Autodesk Fusion 360 part; units mm, degrees
note: some values were not read from the file. Set by a fixed rule: which sketch regions a step uses.
(part 5 of 15)
  line L3455 (261.579, -122.394) -> (261.6, -122.21)
  line L3456 (263.32, -121.881) -> (263.407, -122.045)
  line L3457 (42.9075, -121.723) -> (43.0718, -121.637)
  line L3458 (71.3052, -121.572) -> (71.4695, -121.486)
  line L3459 (70.8754, -122.354) -> (70.8961, -122.17)
  line L3460 (43.0718, -121.637) -> (43.2497, -121.585)
  line L3461 (282.196, -122.153) -> (282.03, -122.236)
  line L3462 (72.7572, -122.183) -> (72.7753, -122.367)
  line L3463 (42.5545, -122.144) -> (42.6438, -121.982)
  line L3464 (282.637, -121.35) -> (282.636, -121.377)
  line L3465 (282.342, -122.038) -> (282.196, -122.153)
  line L3466 (263.479, -122.407) -> (263.479, -122.434)
  line L3467 (72.1689, -123.253) -> (71.9903, -123.303)
  line L3468 (262.009, -121.612) -> (262.173, -121.526)
  line L3469 (71.0268, -122.882) -> (70.9421, -122.717)
  line L3470 (261.6, -122.21) -> (261.656, -122.033)
  line L3471 (72.0164, -121.437) -> (72.1935, -121.491)
  line L3472 (282.636, -121.377) -> (282.613, -121.561)
  line L3473 (261.745, -121.87) -> (261.864, -121.728)
  line L3474 (282.478, -120.825) -> (282.565, -120.988)
  line L3475 (72.4994, -121.698) -> (72.6166, -121.841)
  line L3476 (42.4984, -122.321) -> (42.5545, -122.144)
  line L3477 (72.775, -122.394) -> (72.7517, -122.578)
  line L3478 (72.4805, -123.055) -> (72.3344, -123.169)
  line L3479 (262.149, -123.278) -> (261.987, -123.187)
  line L3480 (262.873, -123.293) -> (262.694, -123.343)
  line L3481 (262.351, -121.474) -> (262.536, -121.457)
  line L3482 (71.8054, -123.317) -> (71.6213, -123.295)
  line L3483 (263.06, -121.62) -> (263.203, -121.738)
  line L3484 (72.3566, -121.58) -> (72.4994, -121.698)
  line L3485 (53.5942, -121.521) -> (53.5357, -121.697)
  line L3486 (53.3419, -120.641) -> (53.4591, -120.785)
  line L3487 (51.7946, -120.936) -> (51.8839, -120.774)
  line L3488 (52.3119, -120.43) -> (52.4898, -120.377)
  line L3489 (51.7845, -121.66) -> (51.7334, -121.482)
  line L3490 (70.8909, -122.539) -> (70.8754, -122.354)
  line L3491 (51.7386, -121.113) -> (51.7946, -120.936)
  line L3492 (52.8328, -122.246) -> (52.6479, -122.26)
  line L3493 (53.5357, -121.697) -> (53.4441, -121.858)
  line L3494 (301.464, -120.006) -> (301.607, -120.125)
  line L3495 (281.022, -120.672) -> (281.167, -120.556)
  line L3496 (52.6479, -122.26) -> (52.4638, -122.238)
  line L3497 (301.607, -120.125) -> (301.724, -120.268)
  line L3498 (282.555, -121.737) -> (282.463, -121.898)
  line L3499 (280.814, -120.976) -> (280.903, -120.814)
  line L3500 (52.8588, -120.38) -> (53.0359, -120.435)
  line L3501 (53.4591, -120.785) -> (53.5461, -120.948)
  line L3502 (281.693, -120.401) -> (281.878, -120.42)
  line L3503 (301.724, -120.268) -> (301.811, -120.432)
  line L3504 (301.864, -120.61) -> (301.882, -120.794)
  line L3505 (281.003, -122.01) -> (280.888, -121.865)
  line L3506 (282.218, -120.563) -> (282.361, -120.681)
  line L3507 (281.331, -120.47) -> (281.509, -120.417)
  line L3508 (51.7179, -121.297) -> (51.7386, -121.113)
  line L3509 (281.483, -122.278) -> (281.306, -122.221)
  line L3510 (51.8693, -121.825) -> (51.7845, -121.66)
  line L3511 (280.737, -121.337) -> (280.757, -121.153)
  line L3512 (52.1476, -120.515) -> (52.3119, -120.43)
  line L3513 (71.832, -121.417) -> (72.0164, -121.437)
  line L3514 (281.509, -120.417) -> (281.693, -120.401)
  line L3515 (280.752, -121.522) -> (280.737, -121.337)
  line L3516 (53.3229, -121.998) -> (53.1768, -122.113)
  line L3517 (280.803, -121.7) -> (280.752, -121.522)
  line L3518 (53.1768, -122.113) -> (53.0113, -122.196)
  line L3519 (52.0031, -120.632) -> (52.1476, -120.515)
  line L3520 (301.859, -121.005) -> (301.8, -121.18)
  line L3521 (53.0113, -122.196) -> (52.8328, -122.246)
  line L3522 (70.9421, -122.717) -> (70.8909, -122.539)
  line L3523 (281.167, -120.556) -> (281.331, -120.47)
  line L3524 (71.0415, -121.83) -> (71.1607, -121.688)
  line L3525 (281.145, -122.131) -> (281.003, -122.01)
  line L3526 (53.5461, -120.948) -> (53.5997, -121.126)
  line L3527 (52.2875, -122.181) -> (52.1256, -122.091)
  line L3528 (71.1607, -121.688) -> (71.3052, -121.572)
  line L3529 (53.6174, -121.337) -> (53.5942, -121.521)
  line L3530 (52.4898, -120.377) -> (52.6744, -120.36)
  line L3531 (280.903, -120.814) -> (281.022, -120.672)
  line L3532 (282.361, -120.681) -> (282.478, -120.825)
  line L3533 (53.6178, -121.31) -> (53.6174, -121.337)
  line L3534 (301.123, -119.863) -> (301.301, -119.918)
  line L3535 (281.306, -122.221) -> (281.145, -122.131)
  line L3536 (52.6744, -120.36) -> (52.8588, -120.38)
  line L3537 (281.667, -122.3) -> (281.483, -122.278)
  line L3538 (282.613, -121.561) -> (282.555, -121.737)
  line L3539 (52.1256, -122.091) -> (51.9844, -121.97)
  line L3540 (301.301, -119.918) -> (301.464, -120.006)
  line L3541 (51.7334, -121.482) -> (51.7179, -121.297)
  line L3542 (70.9522, -121.993) -> (71.0415, -121.83)
  line L3543 (280.757, -121.153) -> (280.814, -120.976)
  line L3544 (53.5997, -121.126) -> (53.6178, -121.31)
  line L3545 (53.0359, -120.435) -> (53.199, -120.523)
  line L3546 (280.888, -121.865) -> (280.803, -121.7)
  line L3547 (53.199, -120.523) -> (53.3419, -120.641)
  line L3548 (53.4441, -121.858) -> (53.3229, -121.998)
  line L3549 (301.442, -121.596) -> (301.276, -121.68)
  line L3550 (34.372, -120.754) -> (34.3717, -120.781)
  line L3551 (300.728, -121.722) -> (300.552, -121.665)
  line L3552 (301.811, -120.432) -> (301.864, -120.61)
  line L3553 (301.8, -121.18) -> (301.709, -121.342)
  line L3554 (52.4638, -122.238) -> (52.2875, -122.181)
  line L3555 (34.2133, -120.228) -> (34.3004, -120.392)
  line L3556 (300.577, -119.913) -> (300.754, -119.861)
  line L3557 (34.2899, -121.14) -> (34.1983, -121.302)
  line L3558 (299.983, -120.781) -> (300.003, -120.597)
  line L3559 (300.754, -119.861) -> (300.939, -119.844)
  line L3560 (300.39, -121.574) -> (300.249, -121.454)
  line L3561 (299.998, -120.966) -> (299.983, -120.781)
  line L3562 (300.913, -121.744) -> (300.728, -121.722)
  line L3563 (32.9018, -119.959) -> (33.0662, -119.873)
  line L3564 (33.587, -121.69) -> (33.4021, -121.704)
  line L3565 (32.5489, -120.38) -> (32.6382, -120.217)
  line L3566 (300.134, -121.309) -> (300.049, -121.144)
  line L3567 (34.0961, -120.085) -> (34.2133, -120.228)
  line L3568 (34.1983, -121.302) -> (34.0772, -121.442)
  line L3569 (32.6235, -121.269) -> (32.5387, -121.104)
  line L3570 (300.412, -119.999) -> (300.577, -119.913)
  line L3571 (199.319, -117.044) -> (199.582, -117.146)
  line L3572 (33.9311, -121.556) -> (33.7656, -121.64)
  line L3573 (33.4287, -119.804) -> (33.6131, -119.823)
  line L3574 (33.7902, -119.878) -> (33.9533, -119.966)
  line L3575 (301.097, -121.73) -> (300.913, -121.744)
  line L3576 (300.059, -120.42) -> (300.149, -120.257)
  line L3577 (200.711, -118.673) -> (200.731, -118.955)
  line L3578 (32.6382, -120.217) -> (32.7574, -120.075)
  line L3579 (300.552, -121.665) -> (300.39, -121.574)
  line L3580 (300.149, -120.257) -> (300.268, -120.115)
  line L3581 (200.419, -117.884) -> (200.553, -118.132)
  line L3582 (200.651, -118.397) -> (200.711, -118.673)
  line L3583 (33.244, -119.821) -> (33.4287, -119.804)
  line L3584 (301.276, -121.68) -> (301.097, -121.73)
  line L3585 (300.049, -121.144) -> (299.998, -120.966)
  line L3586 (34.3004, -120.392) -> (34.3539, -120.569)
  line L3587 (34.3484, -120.964) -> (34.2899, -121.14)
  line L3588 (301.882, -120.794) -> (301.882, -120.821)
  line L3589 (199.829, -117.284) -> (200.053, -117.455)
  line L3590 (199.043, -116.98) -> (199.319, -117.044)
  line L3591 (300.249, -121.454) -> (300.134, -121.309)
  line L3592 (200.553, -118.132) -> (200.651, -118.397)
  line L3593 (33.0662, -119.873) -> (33.244, -119.821)
  line L3594 (51.8839, -120.774) -> (52.0031, -120.632)
  line L3595 (300.939, -119.844) -> (301.123, -119.863)
  line L3596 (301.588, -121.482) -> (301.442, -121.596)
  line L3597 (33.7656, -121.64) -> (33.587, -121.69)
  line L3598 (33.218, -121.682) -> (33.0417, -121.625)
  line L3599 (200.053, -117.455) -> (200.251, -117.656)
  line L3600 (200.251, -117.656) -> (200.419, -117.884)
  line L3601 (32.5387, -121.104) -> (32.4876, -120.925)
  line L3602 (33.9533, -119.966) -> (34.0961, -120.085)
  line L3603 (34.0772, -121.442) -> (33.9311, -121.556)
  line L3604 (300.268, -120.115) -> (300.412, -119.999)
  line L3605 (34.3717, -120.781) -> (34.3484, -120.964)
  line L3606 (33.4021, -121.704) -> (33.218, -121.682)
  line L3607 (51.9844, -121.97) -> (51.8693, -121.825)
  line L3608 (301.882, -120.821) -> (301.859, -121.005)
  line L3609 (34.3539, -120.569) -> (34.372, -120.754)
  line L3610 (33.6131, -119.823) -> (33.7902, -119.878)
  line L3611 (301.709, -121.342) -> (301.588, -121.482)
  line L3612 (300.003, -120.597) -> (300.059, -120.42)
  line L3613 (40.1135, -120.564) -> (40.2477, -120.813)
  line L3614 (38.8917, -123.581) -> (38.6131, -123.627)
  line L3615 (36.4369, -121.856) -> (36.4258, -121.573)
  line L3616 (39.6507, -123.216) -> (39.4158, -123.373)
  line L3617 (36.6288, -120.756) -> (36.7707, -120.512)
  line L3618 (36.5227, -121.018) -> (36.6288, -120.756)
  line L3619 (36.4546, -121.292) -> (36.5227, -121.018)
  line L3620 (36.7707, -120.512) -> (36.9456, -120.29)
  line L3621 (40.2477, -120.813) -> (40.3454, -121.078)
  line L3622 (40.4209, -121.762) -> (40.3833, -122.042)
  line L3623 (39.4158, -123.373) -> (39.1611, -123.496)
  line L3624 (37.0558, -123.094) -> (36.864, -122.887)
  line L3625 (39.1611, -123.496) -> (38.8917, -123.581)
  line L3626 (39.8611, -123.028) -> (39.6507, -123.216)
  line L3627 (271.377, -103.409) -> (271.406, -103.128)
  line L3628 (62.2044, -105.012) -> (61.9695, -105.169)
  line L3629 (275.376, -103.472) -> (275.372, -103.598)
  line L3630 (62.8992, -102.874) -> (62.9587, -103.15)
  line L3631 (272.468, -105.254) -> (272.226, -105.108)
  line L3632 (61.1668, -105.423) -> (60.8844, -105.43)
  line L3633 (273.282, -105.47) -> (273.001, -105.437)
  line L3634 (60.8844, -105.43) -> (60.6039, -105.397)
  line L3635 (273.407, -101.472) -> (273.689, -101.497)
  line L3636 (274.812, -104.864) -> (274.602, -105.052)
  line L3637 (62.8604, -104.109) -> (62.7461, -104.368)
  line L3638 (60.6039, -105.397) -> (60.3308, -105.324)
  line L3639 (62.3012, -101.932) -> (62.4994, -102.133)
  line L3640 (62.8014, -102.609) -> (62.8992, -102.874)
  line L3641 (275.334, -103.878) -> (275.258, -104.15)
  line L3642 (61.2915, -101.457) -> (61.5667, -101.52)
  line L3643 (271.528, -104.237) -> (271.439, -103.969)
  line L3644 (60.0706, -105.214) -> (59.8286, -105.068)
  line L3645 (271.897, -102.126) -> (272.101, -101.931)
  line L3646 (271.406, -103.128) -> (271.474, -102.854)
  line L3647 (275.199, -102.649) -> (275.296, -102.914)
  line L3648 (271.439, -103.969) -> (271.388, -103.692)
  line L3649 (271.474, -102.854) -> (271.58, -102.592)
  line L3650 (271.722, -102.348) -> (271.897, -102.126)
  line L3651 (274.112, -105.332) -> (273.843, -105.417)
  line L3652 (61.4455, -105.377) -> (61.1668, -105.423)
  line L3653 (-67.7892, -104.36) -> (-67.6114, -104.307)
  line L3654 (271.654, -104.49) -> (271.528, -104.237)
  line L3655 (274.602, -105.052) -> (274.367, -105.209)
  line L3656 (62.7461, -104.368) -> (62.5966, -104.608)
  line L3657 (62.6673, -102.36) -> (62.8014, -102.609)
  line L3658 (272.848, -101.543) -> (273.125, -101.488)
  line L3659 (272.331, -101.767) -> (272.582, -101.637)
  line L3660 (274.994, -104.648) -> (274.812, -104.864)
  line L3661 (-68.2319, -105.755) -> (-68.3166, -105.59)
  line L3662 (272.007, -104.93) -> (271.815, -104.723)
  line L3663 (273.001, -105.437) -> (272.728, -105.364)
  line L3664 (62.9786, -103.432) -> (62.9747, -103.558)
  line L3665 (273.125, -101.488) -> (273.407, -101.472)
  line L3666 (60.3308, -105.324) -> (60.0706, -105.214)
  line L3667 (62.5966, -104.608) -> (62.4149, -104.824)
  line L3668 (271.58, -102.592) -> (271.722, -102.348)
  line L3669 (62.4994, -102.133) -> (62.6673, -102.36)
  line L3670 (272.728, -105.364) -> (272.468, -105.254)
  line L3671 (271.388, -103.692) -> (271.377, -103.409)
  line L3672 (275.356, -103.19) -> (275.376, -103.472)
  line L3673 (273.564, -105.463) -> (273.282, -105.47)
  line L3674 (275.258, -104.15) -> (275.143, -104.408)
  line L3675 (272.226, -105.108) -> (272.007, -104.93)
  line L3676 (275.143, -104.408) -> (274.994, -104.648)
  line L3677 (62.0767, -101.76) -> (62.3012, -101.932)
  line L3678 (275.372, -103.598) -> (275.334, -103.878)
  line L3679 (61.7149, -105.292) -> (61.4455, -105.377)
  line L3680 (271.815, -104.723) -> (271.654, -104.49)
  line L3681 (-68.2172, -104.704) -> (-68.098, -104.562)
  line L3682 (274.367, -105.209) -> (274.112, -105.332)
  line L3683 (275.296, -102.914) -> (275.356, -103.19)
  line L3684 (61.5667, -101.52) -> (61.8302, -101.622)
  line L3685 (273.843, -105.417) -> (273.564, -105.463)
  line L3686 (62.9587, -103.15) -> (62.9786, -103.432)
  line L3687 (272.101, -101.931) -> (272.331, -101.767)
  line L3688 (62.4149, -104.824) -> (62.2044, -105.012)
  line L3689 (62.9371, -103.838) -> (62.8604, -104.109)
  line L3690 (61.9695, -105.169) -> (61.7149, -105.292)
  line L3691 (61.8302, -101.622) -> (62.0767, -101.76)
  line L3692 (272.582, -101.637) -> (272.848, -101.543)
  line L3693 (62.9747, -103.558) -> (62.9371, -103.838)
  line L3694 (58.9907, -103.651) -> (58.9796, -103.369)
  line L3695 (59.1309, -104.197) -> (59.0414, -103.929)
  line L3696 (-67.0898, -106.126) -> (-67.2684, -106.176)
  line L3697 (-66.4837, -105.267) -> (-66.507, -105.451)
  line L3698 (-66.6571, -105.788) -> (-66.7782, -105.929)
  line L3699 (-67.9755, -106.021) -> (-68.1167, -105.9)
  line L3700 (-67.6373, -106.168) -> (-67.8137, -106.111)
  line L3701 (-67.8137, -106.111) -> (-67.9755, -106.021)
  line L3702 (-68.1167, -105.9) -> (-68.2319, -105.755)
  line L3703 (-67.9535, -104.446) -> (-67.7892, -104.36)
  line L3704 (-66.5655, -105.627) -> (-66.6571, -105.788)
  line L3705 (256.587, -84.2166) -> (256.704, -84.3603)
  line L3706 (49.6633, -85.8676) -> (49.5015, -85.7772)
  line L3707 (49.5015, -85.7772) -> (49.3603, -85.657)
  line L3708 (256.84, -85.0965) -> (256.781, -85.2724)
  line L3709 (255.371, -85.6661) -> (255.23, -85.546)
  line L3710 (255.03, -85.2358) -> (254.979, -85.0575)
  line L3711 (50.5527, -85.7992) -> (50.3872, -85.8828)
  line L3712 (256.781, -85.2724) -> (256.689, -85.4337)
  line L3713 (256.281, -84.0103) -> (256.444, -84.0985)
  line L3714 (254.963, -84.8728) -> (254.984, -84.6885)
  line L3715 (50.8349, -84.4713) -> (50.922, -84.6351)
  line L3716 (254.979, -85.0575) -> (254.963, -84.8728)
  line L3717 (256.104, -83.9554) -> (256.281, -84.0103)
  line L3718 (256.863, -84.886) -> (256.863, -84.9126)
  line L3719 (256.863, -84.9126) -> (256.84, -85.0965)
  line L3720 (50.0503, -84.0471) -> (50.2347, -84.0665)
  line L3721 (255.23, -85.546) -> (255.115, -85.4007)
  line L3722 (256.689, -85.4337) -> (256.568, -85.574)
  line L3723 (283.791, -84.2422) -> (283.955, -84.1563)
  line L3724 (50.2347, -84.0665) -> (50.4118, -84.1213)
  line L3725 (254.984, -84.6885) -> (255.04, -84.5118)
  line L3726 (49.6878, -84.1162) -> (49.8657, -84.0639)
  line L3727 (255.115, -85.4007) -> (255.03, -85.2358)
  line L3728 (255.893, -85.8358) -> (255.709, -85.8139)
  line L3729 (284.133, -84.104) -> (284.317, -84.0872)
  line L3730 (255.533, -85.7566) -> (255.371, -85.6661)
  line L3731 (50.4118, -84.1213) -> (50.5749, -84.2095)
  line L3732 (256.704, -84.3603) -> (256.791, -84.524)
  line L3733 (255.709, -85.8139) -> (255.533, -85.7566)
  line L3734 (283.646, -84.3584) -> (283.791, -84.2422)
  line L3735 (50.5749, -84.2095) -> (50.7178, -84.3277)
  line L3736 (50.0238, -85.9469) -> (49.8397, -85.9249)
  line L3737 (49.3603, -85.657) -> (49.2451, -85.5117)
  line L3738 (49.1705, -84.6228) -> (49.2598, -84.4603)
  line L3739 (49.8657, -84.0639) -> (50.0503, -84.0471)
  line L3740 (49.2598, -84.4603) -> (49.379, -84.3183)
  line L3741 (256.568, -85.574) -> (256.422, -85.6882)
  line L3742 (50.9701, -85.2075) -> (50.9115, -85.3835)
  line L3743 (50.9937, -84.9971) -> (50.9933, -85.0236)
  line L3744 (50.82, -85.5447) -> (50.6988, -85.685)
  line L3745 (49.5235, -84.2021) -> (49.6878, -84.1162)
  line L3746 (256.078, -85.8216) -> (255.893, -85.8358)
  line L3747 (49.1093, -85.1686) -> (49.0938, -84.9838)
  line L3748 (256.422, -85.6882) -> (256.257, -85.7717)
  line L3749 (255.248, -84.2073) -> (255.393, -84.0911)
  line L3750 (49.1144, -84.7996) -> (49.1705, -84.6228)
  line L3751 (79.2176, -85.3936) -> (79.0965, -85.5339)
  line L3752 (256.257, -85.7717) -> (256.078, -85.8216)
  line L3753 (49.1604, -85.3468) -> (49.1093, -85.1686)
  line L3754 (50.6988, -85.685) -> (50.5527, -85.7992)
  line L3755 (50.9115, -85.3835) -> (50.82, -85.5447)
  line L3756 (49.2451, -85.5117) -> (49.1604, -85.3468)
  line L3757 (49.8397, -85.9249) -> (49.6633, -85.8676)
  line L3758 (50.7178, -84.3277) -> (50.8349, -84.4713)
  line L3759 (50.9933, -85.0236) -> (50.9701, -85.2075)
  line L3760 (50.2086, -85.9326) -> (50.0238, -85.9469)
  line L3761 (284.317, -84.0872) -> (284.502, -84.1065)
  line L3762 (49.379, -84.3183) -> (49.5235, -84.2021)
  line L3763 (256.791, -84.524) -> (256.845, -84.7015)
  line L3764 (256.444, -84.0985) -> (256.587, -84.2166)
  line L3765 (49.0938, -84.9838) -> (49.1144, -84.7996)
  line L3766 (283.955, -84.1563) -> (284.133, -84.104)
  line L3767 (50.3872, -85.8828) -> (50.2086, -85.9326)
  line L3768 (256.845, -84.7015) -> (256.863, -84.886)
  line L3769 (78.9726, -84.0584) -> (79.1154, -84.1766)
  line L3770 (77.8992, -85.6261) -> (77.758, -85.5059)
  line L3771 (79.3092, -85.2324) -> (79.2176, -85.3936)
  line L3772 (78.6063, -85.7815) -> (78.4214, -85.7958)
  line L3773 (77.4914, -84.8327) -> (77.5121, -84.6485)
  line L3774 (255.92, -83.9361) -> (256.104, -83.9554)
  line L3775 (78.2373, -85.7738) -> (78.061, -85.7165)
  line L3776 (255.557, -84.0052) -> (255.735, -83.9529)
  line L3777 (78.6324, -83.9154) -> (78.8095, -83.9702)
  line L3778 (255.129, -84.3493) -> (255.248, -84.2073)
  line L3779 (78.0855, -83.9651) -> (78.2633, -83.9128)
  line L3780 (78.7849, -85.7317) -> (78.6063, -85.7815)
  line L3781 (276.02, -83.8558) -> (275.997, -84.0398)
  line L3782 (79.0965, -85.5339) -> (78.9504, -85.6481)
  line L3783 (77.758, -85.5059) -> (77.6428, -85.3606)
  line L3784 (79.3732, -84.6615) -> (79.3913, -84.846)
  line L3785 (274.529, -84.6094) -> (274.387, -84.4892)
  line L3786 (255.393, -84.0911) -> (255.557, -84.0052)
  line L3787 (79.3197, -84.484) -> (79.3732, -84.6615)
  line L3788 (77.6428, -85.3606) -> (77.558, -85.1957)
  line L3789 (275.862, -83.3036) -> (275.949, -83.4673)
  line L3790 (77.5121, -84.6485) -> (77.5682, -84.4717)
  line L3791 (78.2633, -83.9128) -> (78.448, -83.896)
  line L3792 (79.3913, -84.846) -> (79.391, -84.8725)
  line L3793 (275.949, -83.4673) -> (276.003, -83.6448)
  line L3794 (78.4214, -85.7958) -> (78.2373, -85.7738)
  line L3795 (79.1154, -84.1766) -> (79.2326, -84.3203)
  line L3796 (78.061, -85.7165) -> (77.8992, -85.6261)
  line L3797 (255.735, -83.9529) -> (255.92, -83.9361)
  line L3798 (79.2326, -84.3203) -> (79.3197, -84.484)
  line L3799 (275.847, -84.3769) -> (275.726, -84.5173)
  line L3800 (274.387, -84.4892) -> (274.272, -84.3439)
  line L3801 (275.939, -84.2157) -> (275.847, -84.3769)
  line L3802 (78.9504, -85.6481) -> (78.7849, -85.7317)
  line L3803 (79.391, -84.8725) -> (79.3677, -85.0564)
  line L3804 (274.272, -84.3439) -> (274.187, -84.179)
  line L3805 (275.745, -83.1599) -> (275.862, -83.3036)
  line L3806 (275.726, -84.5173) -> (275.58, -84.6314)
  line L3807 (276.021, -83.8293) -> (276.02, -83.8558)
  line L3808 (275.58, -84.6314) -> (275.414, -84.715)
  line L3809 (77.5069, -85.0175) -> (77.4914, -84.8327)
  line L3810 (77.558, -85.1957) -> (77.5069, -85.0175)
  line L3811 (274.187, -84.179) -> (274.136, -84.0008)
  line L3812 (274.136, -84.0008) -> (274.121, -83.816)
  line L3813 (255.04, -84.5118) -> (255.129, -84.3493)
  line L3814 (275.602, -83.0417) -> (275.745, -83.1599)
  line L3815 (79.3677, -85.0564) -> (79.3092, -85.2324)
  line L3816 (78.8095, -83.9702) -> (78.9726, -84.0584)
  line L3817 (275.414, -84.715) -> (275.236, -84.7649)
  line L3818 (60.2157, -83.6047) -> (60.2338, -83.7892)
  line L3819 (60.2334, -83.8158) -> (60.2102, -83.9997)
  line L3820 (274.867, -84.7572) -> (274.69, -84.6999)
  line L3821 (274.69, -84.6999) -> (274.529, -84.6094)
  line L3822 (274.287, -83.2926) -> (274.406, -83.1506)
  line L3823 (77.6575, -84.3093) -> (77.7767, -84.1672)
  line L3824 (59.7928, -84.5914) -> (59.6273, -84.675)
  line L3825 (59.4488, -84.7248) -> (59.2639, -84.739)
  line L3826 (59.0798, -84.7171) -> (58.9035, -84.6598)
  line L3827 (58.4853, -84.3039) -> (58.4005, -84.139)
  line L3828 (59.2639, -84.739) -> (59.0798, -84.7171)
  line L3829 (60.1517, -84.1756) -> (60.0601, -84.3369)
  line L3830 (274.121, -83.816) -> (274.141, -83.6318)
  line L3831 (59.9579, -83.1198) -> (60.0751, -83.2635)
  line L3832 (59.815, -83.0017) -> (59.9579, -83.1198)
  line L3833 (275.077, -82.8793) -> (275.262, -82.8987)
  line L3834 (274.893, -82.8961) -> (275.077, -82.8793)
  line L3835 (59.6273, -84.675) -> (59.4488, -84.7248)
  line L3836 (58.9035, -84.6598) -> (58.7416, -84.5693)
  line L3837 (274.198, -83.4551) -> (274.287, -83.2926)
  line L3838 (58.3339, -83.776) -> (58.3545, -83.5917)
  line L3839 (58.9279, -82.9084) -> (59.1058, -82.8561)
  line L3840 (58.6191, -83.1105) -> (58.7636, -82.9943)
  line L3841 (58.7416, -84.5693) -> (58.6004, -84.4492)
  line L3842 (78.448, -83.896) -> (78.6324, -83.9154)
  line L3843 (274.551, -83.0344) -> (274.715, -82.9485)
  line L3844 (295.108, -82.7471) -> (295.195, -82.9108)
  line L3845 (58.4999, -83.2525) -> (58.6191, -83.1105)
  line L3846 (294.66, -84.1586) -> (294.481, -84.2084)
  line L3847 (274.406, -83.1506) -> (274.551, -83.0344)
  line L3848 (60.1621, -83.4272) -> (60.2157, -83.6047)
  line L3849 (274.141, -83.6318) -> (274.198, -83.4551)
  line L3850 (58.4005, -84.139) -> (58.3494, -83.9607)
  line L3851 (295.093, -83.8205) -> (294.972, -83.9608)
  line L3852 (295.195, -82.9108) -> (295.248, -83.0883)
  line L3853 (59.9389, -84.4772) -> (59.7928, -84.5914)
  line L3854 (294.972, -83.9608) -> (294.826, -84.075)
  line L3855 (58.7636, -82.9943) -> (58.9279, -82.9084)
  line L3856 (275.439, -82.9535) -> (275.602, -83.0417)
  line L3857 (77.9212, -84.051) -> (78.0855, -83.9651)
  line L3858 (275.236, -84.7649) -> (275.051, -84.7791)
  line L3859 (60.2102, -83.9997) -> (60.1517, -84.1756)
  line L3860 (60.2338, -83.7892) -> (60.2334, -83.8158)
  line L3861 (58.6004, -84.4492) -> (58.4853, -84.3039)
  line L3862 (274.715, -82.9485) -> (274.893, -82.8961)
  line L3863 (60.0601, -84.3369) -> (59.9389, -84.4772)
  line L3864 (58.3545, -83.5917) -> (58.4106, -83.415)
  line L3865 (60.0751, -83.2635) -> (60.1621, -83.4272)
  line L3866 (59.6519, -82.9135) -> (59.815, -83.0017)
  line L3867 (295.184, -83.6593) -> (295.093, -83.8205)
  line L3868 (294.826, -84.075) -> (294.66, -84.1586)
  line L3869 (294.481, -84.2084) -> (294.297, -84.2227)
  line L3870 (295.243, -83.4833) -> (295.184, -83.6593)
  line L3871 (59.4748, -82.8587) -> (59.6519, -82.9135)
  line L3872 (294.297, -84.2227) -> (294.112, -84.2007)
  line L3873 (58.4106, -83.415) -> (58.4999, -83.2525)
  line L3874 (58.3494, -83.9607) -> (58.3339, -83.776)
  line L3875 (275.262, -82.8987) -> (275.439, -82.9535)
  line L3876 (77.7767, -84.1672) -> (77.9212, -84.051)
  line L3877 (276.003, -83.6448) -> (276.021, -83.8293)
  line L3878 (275.997, -84.0398) -> (275.939, -84.2157)
  line L3879 (275.051, -84.7791) -> (274.867, -84.7572)
  line L3880 (77.5682, -84.4717) -> (77.6575, -84.3093)
  line L3881 (40.7121, -82.5634) -> (40.8293, -82.7071)
  line L3882 (295.248, -83.0883) -> (295.266, -83.2729)
  line L3883 (39.6577, -84.1033) -> (39.4958, -84.0129)
  line L3884 (39.4958, -84.0129) -> (39.3547, -83.8927)
  line L3885 (293.936, -84.1434) -> (293.774, -84.053)
  line L3886 (293.961, -82.392) -> (294.138, -82.3397)
  line L3887 (-47.0692, -80.808) -> (-46.9098, -81.0239)
  line L3888 (40.9877, -83.2593) -> (40.9644, -83.4433)
  line L3889 (59.2904, -82.8393) -> (59.4748, -82.8587)
  line L3890 (293.387, -83.0754) -> (293.443, -82.8986)
  line L3891 (40.5693, -82.4452) -> (40.7121, -82.5634)
  line L3892 (-47.1496, -83.3642) -> (-47.3495, -83.5433)
  line L3893 (-47.705, -80.3228) -> (-47.4709, -80.454)
  line L3894 (39.834, -84.1606) -> (39.6577, -84.1033)
  line L3895 (39.1036, -83.4043) -> (39.0881, -83.2195)
  line L3896 (294.991, -82.6035) -> (295.108, -82.7471)
  line L3897 (40.8143, -83.7804) -> (40.6932, -83.9208)
  line L3898 (294.138, -82.3397) -> (294.323, -82.3229)
  line L3899 (-47.4709, -80.454) -> (-47.2575, -80.6168)
  line L3900 (39.5178, -82.4379) -> (39.6822, -82.352)
  line L3901 (59.1058, -82.8561) -> (59.2904, -82.8393)
  line L3902 (294.112, -84.2007) -> (293.936, -84.1434)
  line L3903 (40.6932, -83.9208) -> (40.5471, -84.0349)
  line L3904 (293.533, -82.7361) -> (293.652, -82.5941)
  line L3905 (294.685, -82.3971) -> (294.848, -82.4853)
  line L3906 (-46.633, -81.7743) -> (-46.614, -82.042)
  line L3907 (293.518, -83.7875) -> (293.433, -83.6226)
  line L3908 (39.3547, -83.8927) -> (39.2395, -83.7474)
  line L3909 (293.774, -84.053) -> (293.633, -83.9328)
  line L3910 (40.9644, -83.4433) -> (40.9059, -83.6192)
  line L3911 (294.848, -82.4853) -> (294.991, -82.6035)
  line L3912 (40.5471, -84.0349) -> (40.3816, -84.1185)
  line L3913 (40.9699, -83.0483) -> (40.988, -83.2328)
  line L3914 (293.652, -82.5941) -> (293.796, -82.4779)
  line L3915 (-46.6177, -82.1613) -> (-46.6535, -82.4273)
  line L3916 (39.1547, -83.5825) -> (39.1036, -83.4043)
  line L3917 (-47.5726, -83.6924) -> (-47.8146, -83.8086)
  line L3918 (293.382, -83.4444) -> (293.367, -83.2596)
  line L3919 (40.4062, -82.357) -> (40.5693, -82.4452)
  line L3920 (294.508, -82.3423) -> (294.685, -82.3971)
  line L3921 (295.266, -83.2994) -> (295.243, -83.4833)
  line L3922 (293.796, -82.4779) -> (293.961, -82.392)
  line L3923 (-47.3495, -83.5433) -> (-47.5726, -83.6924)
  line L3924 (-46.6894, -81.5119) -> (-46.633, -81.7743)
  line L3925 (40.3816, -84.1185) -> (40.203, -84.1684)
  line L3926 (40.9059, -83.6192) -> (40.8143, -83.7804)
  line L3927 (293.367, -83.2596) -> (293.387, -83.0754)
  line L3928 (40.988, -83.2328) -> (40.9877, -83.2593)
  line L3929 (39.3733, -82.5541) -> (39.5178, -82.4379)
  line L3930 (39.2395, -83.7474) -> (39.1547, -83.5825)
  line L3931 (293.633, -83.9328) -> (293.518, -83.7875)
  line L3932 (-47.9553, -80.226) -> (-47.705, -80.3228)
  line L3933 (295.266, -83.2729) -> (295.266, -83.2994)
  line L3934 (-46.9098, -81.0239) -> (-46.7823, -81.2601)
  line L3935 (-46.614, -82.042) -> (-46.6177, -82.1613)
  line L3936 (-47.8146, -83.8086) -> (-48.0705, -83.8895)
  line L3937 (293.443, -82.8986) -> (293.533, -82.7361)
  line L3938 (40.9163, -82.8708) -> (40.9699, -83.0483)
  line L3939 (293.433, -83.6226) -> (293.382, -83.4444)
  line L3940 (40.2291, -82.3022) -> (40.4062, -82.357)
  line L3941 (40.203, -84.1684) -> (40.0181, -84.1826)
  line L3942 (40.0181, -84.1826) -> (39.834, -84.1606)
  line L3943 (294.323, -82.3229) -> (294.508, -82.3423)
  line L3944 (40.8293, -82.7071) -> (40.9163, -82.8708)
  line L3945 (193.803, -80.3625) -> (193.937, -80.6111)
  line L3946 (-48.87, -83.9083) -> (-49.1294, -83.8396)
  line L3947 (-49.5067, -80.422) -> (-49.2686, -80.2983)
  line L3948 (-50.4025, -82.2505) -> (-50.4131, -81.9823)
  line L3949 (-50.0855, -80.974) -> (-49.9193, -80.7633)
  line L3950 (-48.0705, -83.8895) -> (-48.3352, -83.9336)
  line L3951 (-46.6535, -82.4273) -> (-46.7263, -82.6856)
  line L3952 (190.267, -82.1995) -> (190.177, -81.9315)
  line L3953 (-50.1494, -83.0092) -> (-50.2694, -82.7691)
  line L3954 (192.703, -79.5225) -> (192.966, -79.6245)
  line L3955 (-48.6035, -83.9399) -> (-48.87, -83.9083)
  line L3956 (-49.6065, -83.5965) -> (-49.8146, -83.427)
  line L3957 (193.882, -82.37) -> (193.733, -82.6097)
  line L3958 (190.745, -82.8921) -> (190.554, -82.6846)
  line L3959 (39.2542, -82.6961) -> (39.3733, -82.5541)
  line L3960 (-50.2203, -81.2061) -> (-50.0855, -80.974)
  line L3961 (-50.3857, -81.7153) -> (-50.321, -81.4549)
  line L3962 (-47.2575, -80.6168) -> (-47.0692, -80.808)
  line L3963 (39.0881, -83.2195) -> (39.1088, -83.0353)
  line L3964 (39.6822, -82.352) -> (39.86, -82.2996)
  line L3965 (-49.1294, -83.8396) -> (-49.3766, -83.7349)
  line L3966 (193.635, -80.1352) -> (193.803, -80.3625)
  line L3967 (193.551, -82.8259) -> (193.34, -83.0144)
  line L3968 (191.207, -83.2161) -> (190.964, -83.0704)
  line L3969 (40.0447, -82.2828) -> (40.2291, -82.3022)
  line L3970 (190.127, -81.6536) -> (190.115, -81.3713)
  line L3971 (192.02, -83.4319) -> (191.74, -83.3987)
  line L3972 (194.115, -81.4341) -> (194.111, -81.5597)
  line L3973 (-49.7251, -80.578) -> (-49.5067, -80.422)
  line L3974 (193.213, -79.7625) -> (193.437, -79.9339)
  line L3975 (39.1648, -82.8586) -> (39.2542, -82.6961)
  line L3976 (39.86, -82.2996) -> (40.0447, -82.2828)
  line L3977 (-46.9769, -83.1588) -> (-47.1496, -83.3642)
  line L3978 (192.427, -79.4587) -> (192.703, -79.5225)
  line L3979 (192.966, -79.6245) -> (193.213, -79.7625)
  line L3980 (-50.3543, -82.5145) -> (-50.4025, -82.2505)
  line L3981 (-48.2168, -80.1654) -> (-47.9553, -80.226)
  line L3982 (-50.4131, -81.9823) -> (-50.3857, -81.7153)
  line L3983 (190.115, -81.3713) -> (190.144, -81.0903)
  line L3984 (-49.2686, -80.2983) -> (-49.0154, -80.2093)
  line L3985 (190.144, -81.0903) -> (190.212, -80.8161)
  line L3986 (194.111, -81.5597) -> (194.073, -81.8397)
  line L3987 (193.34, -83.0144) -> (193.105, -83.1714)
  line L3988 (39.1088, -83.0353) -> (39.1648, -82.8586)
  line L3989 (191.467, -83.3263) -> (191.207, -83.2161)
  line L3990 (-49.3766, -83.7349) -> (-49.6065, -83.5965)
  line L3991 (-49.9193, -80.7633) -> (-49.7251, -80.578)
  line L3992 (-48.4842, -80.1422) -> (-48.2168, -80.1654)
  line L3993 (-46.7263, -82.6856) -> (-46.8348, -82.9311)
  line L3994 (193.437, -79.9339) -> (193.635, -80.1352)
  line L3995 (192.851, -83.2937) -> (192.581, -83.3789)
  line L3996 (192.581, -83.3789) -> (192.303, -83.4252)
  line L3997 (190.177, -81.9315) -> (190.127, -81.6536)
  line L3998 (190.318, -80.5542) -> (190.46, -80.31)
  line L3999 (-49.9968, -83.23) -> (-50.1494, -83.0092)
  line L4000 (190.46, -80.31) -> (190.635, -80.0881)
  line L4001 (-49.0154, -80.2093) -> (-48.7521, -80.157)
  line L4002 (-50.2694, -82.7691) -> (-50.3543, -82.5145)
  line L4003 (-49.8146, -83.427) -> (-49.9968, -83.23)
  line L4004 (-48.7521, -80.157) -> (-48.4842, -80.1422)
  line L4005 (-46.8348, -82.9311) -> (-46.9769, -83.1588)
  line L4006 (-46.7823, -81.2601) -> (-46.6894, -81.5119)
  line L4007 (-48.3352, -83.9336) -> (-48.6035, -83.9399)
  line L4008 (-50.321, -81.4549) -> (-50.2203, -81.2061)
  line L4009 (143.338, -79.7224) -> (143.563, -79.8938)
  line L4010 (144.063, -80.571) -> (144.161, -80.8361)
  line L4011 (144.008, -82.3299) -> (143.858, -82.5696)
  line L4012 (190.554, -82.6846) -> (190.393, -82.4522)
  line L4013 (193.105, -83.1714) -> (192.851, -83.2937)
  line L4014 (144.198, -81.7996) -> (144.122, -82.0715)
  line L4015 (191.74, -83.3987) -> (191.467, -83.3263)
  line L4016 (191.07, -79.7288) -> (191.32, -79.5986)
  line L4017 (191.864, -79.4499) -> (192.146, -79.4344)
  line L4018 (143.929, -80.3224) -> (144.063, -80.571)
  line L4019 (191.587, -79.505) -> (191.864, -79.4499)
  line L4020 (144.24, -81.3941) -> (144.236, -81.5196)
  line L4021 (229.706, -74.5116) -> (229.427, -74.558)
  line L4022 (227.251, -72.7863) -> (227.24, -72.504)
  line L4023 (191.32, -79.5986) -> (191.587, -79.505)
  line L4024 (230.465, -74.1472) -> (230.23, -74.3041)
  line L4025 (229.145, -74.5646) -> (228.864, -74.5314)
  line L4026 (144.236, -81.5196) -> (144.198, -81.7996)
  line L4027 (228.864, -74.5314) -> (228.591, -74.459)
  line L4028 (143.092, -79.5844) -> (143.338, -79.7224)
  line L4029 (142.976, -83.2536) -> (142.707, -83.3388)
  line L4030 (142.553, -79.4187) -> (142.828, -79.4825)
  line L4031 (144.161, -80.8361) -> (144.22, -81.1123)
  line L4032 (143.466, -82.9744) -> (143.231, -83.1313)
  line L4033 (228.988, -70.5826) -> (229.27, -70.5671)
  line L4034 (194.035, -80.8761) -> (194.095, -81.1523)
  line L4035 (143.231, -83.1313) -> (142.976, -83.2536)
  line L4036 (229.27, -70.5671) -> (229.552, -70.5915)
  line L4037 (229.975, -74.4264) -> (229.706, -74.5116)
  line L4038 (227.337, -71.9488) -> (227.443, -71.687)
  line L4039 (105.967, -70.7171) -> (106.214, -70.8552)
  line L4040 (228.711, -70.6377) -> (228.988, -70.5826)
  line L4041 (227.443, -71.687) -> (227.585, -71.4427)
  line L4042 (105.704, -70.6152) -> (105.967, -70.7171)
  line L4043 (227.391, -73.3322) -> (227.302, -73.0642)
  line L4044 (229.427, -74.558) -> (229.145, -74.5646)
  line L4045 (192.146, -79.4344) -> (192.427, -79.4587)
  line L4046 (228.089, -74.2032) -> (227.87, -74.0248)
  line L4047 (144.122, -82.0715) -> (144.008, -82.3299)
  line L4048 (192.303, -83.4252) -> (192.02, -83.4319)
  line L4049 (190.964, -83.0704) -> (190.745, -82.8921)
  line L4050 (194.073, -81.8397) -> (193.996, -82.1116)
  line L4051 (227.759, -71.2208) -> (227.964, -71.0258)
  line L4052 (105.429, -70.5514) -> (105.704, -70.6152)
  line L4053 (106.214, -70.8552) -> (106.438, -71.0266)
  line L4054 (190.212, -80.8161) -> (190.318, -80.5542)
  line L4055 (190.84, -79.8931) -> (191.07, -79.7288)
  line L4056 (227.302, -73.0642) -> (227.251, -72.7863)
  line L4057 (142.828, -79.4825) -> (143.092, -79.5844)
  line L4058 (228.194, -70.8616) -> (228.444, -70.7313)
  line L4059 (227.87, -74.0248) -> (227.678, -73.8173)
  line L4060 (143.563, -79.8938) -> (143.761, -80.0952)
  line L4061 (143.676, -82.7859) -> (143.466, -82.9744)
  line L4062 (144.22, -81.1123) -> (144.24, -81.3941)
  line L4063 (227.24, -72.504) -> (227.269, -72.223)
  line L4064 (143.858, -82.5696) -> (143.676, -82.7859)
  line L4065 (227.585, -71.4427) -> (227.759, -71.2208)
  line L4066 (143.761, -80.0952) -> (143.929, -80.3224)
  line L4067 (193.733, -82.6097) -> (193.551, -82.8259)
  line L4068 (193.996, -82.1116) -> (193.882, -82.37)
  line L4069 (190.635, -80.0881) -> (190.84, -79.8931)
  line L4070 (190.393, -82.4522) -> (190.267, -82.1995)
  line L4071 (193.937, -80.6111) -> (194.035, -80.8761)
  line L4072 (194.095, -81.1523) -> (194.115, -81.4341)
  line L4073 (106.29, -91.3746) -> (106.455, -91.2887)
  line L4074 (-38.3659, -90.7957) -> (-38.4035, -91.0757)
  line L4075 (-38.4802, -91.3476) -> (-38.5944, -91.6059)
  line L4076 (-42.3609, -90.6073) -> (-42.3322, -90.3262)
  line L4077 (-41.0098, -92.5623) -> (-41.2699, -92.4521)
  line L4078 (-38.7439, -91.8457) -> (-38.9257, -92.0619)
  line L4079 (-40.4561, -92.6679) -> (-40.7367, -92.6347)
  line L4080 (-42.0161, -89.5459) -> (-41.8412, -89.3241)
  line L4081 (-41.8412, -89.3241) -> (-41.6368, -89.1291)
  line L4082 (107.761, -92.1695) -> (107.76, -92.196)
  line L4083 (-39.0393, -89.1699) -> (-38.8411, -89.3712)
  line L4084 (107.737, -92.38) -> (107.678, -92.5559)
  line L4085 (105.937, -91.7953) -> (106.027, -91.6328)
  line L4086 (106.43, -93.0401) -> (106.268, -92.9496)
  line L4087 (-42.2097, -91.4355) -> (-42.2991, -91.1675)
  line L4088 (106.455, -91.2887) -> (106.633, -91.2363)
  line L4089 (-38.3819, -90.3883) -> (-38.3619, -90.6701)
  line L4090 (-42.3499, -90.8896) -> (-42.3609, -90.6073)
  line L4091 (-39.2639, -88.9985) -> (-39.0393, -89.1699)
  line L4092 (106.791, -93.1193) -> (106.607, -93.0973)
  line L4093 (-39.7739, -88.7585) -> (-39.5104, -88.8604)
  line L4094 (-38.8411, -89.3712) -> (-38.6733, -89.5984)
  line L4095 (106.146, -91.4908) -> (106.29, -91.3746)
  line L4096 (-38.6733, -89.5984) -> (-38.5391, -89.8471)
  line L4097 (106.127, -92.8294) -> (106.012, -92.6841)
  line L4098 (-42.0834, -91.6882) -> (-42.2097, -91.4355)
  line L4099 (106.027, -91.6328) -> (106.146, -91.4908)
  line L4100 (-39.5104, -88.8604) -> (-39.2639, -88.9985)
  line L4101 (-40.0491, -88.6947) -> (-39.7739, -88.7585)
  line L4102 (-39.6257, -92.5296) -> (-39.895, -92.6148)
  line L4103 (-41.731, -92.128) -> (-41.9228, -91.9206)
  line L4104 (-42.2991, -91.1675) -> (-42.3499, -90.8896)
  line L4105 (-42.264, -90.0521) -> (-42.158, -89.7902)
  line L4106 (105.861, -92.1562) -> (105.881, -91.972)
  line L4107 (106.633, -91.2363) -> (106.817, -91.2195)
  line L4108 (105.876, -92.341) -> (105.861, -92.1562)
  line L4109 (-39.895, -92.6148) -> (-40.1737, -92.6612)
  line L4110 (-42.158, -89.7902) -> (-42.0161, -89.5459)
  line L4111 (-38.9257, -92.0619) -> (-39.1361, -92.2504)
  line L4112 (-42.3322, -90.3262) -> (-42.264, -90.0521)
  line L4113 (107.76, -92.196) -> (107.737, -92.38)
  line L4114 (226.879, -91.5308) -> (227.024, -91.4146)
  line L4115 (227.024, -91.4146) -> (227.188, -91.3287)
  line L4116 (227.002, -92.9897) -> (226.861, -92.8695)
  line L4117 (105.881, -91.972) -> (105.937, -91.7953)
  line L4118 (106.268, -92.9496) -> (106.127, -92.8294)
  line L4119 (-38.5391, -89.8471) -> (-38.4413, -90.1121)
  line L4120 (106.607, -93.0973) -> (106.43, -93.0401)
  line L4121 (106.976, -93.1051) -> (106.791, -93.1193)
  line L4122 (-38.3619, -90.6701) -> (-38.3659, -90.7957)
  line L4123 (106.012, -92.6841) -> (105.927, -92.5192)
  line L4124 (-41.2699, -92.4521) -> (-41.5119, -92.3064)
  line L4125 (-41.9228, -91.9206) -> (-42.0834, -91.6882)
  line L4126 (-38.4035, -91.0757) -> (-38.4802, -91.3476)
  line L4127 (-41.5119, -92.3064) -> (-41.731, -92.128)
  line L4128 (106.817, -91.2195) -> (107.002, -91.2389)
  line L4129 (-38.4413, -90.1121) -> (-38.3819, -90.3883)
  line L4130 (105.927, -92.5192) -> (105.876, -92.341)
  line L4131 (-41.6368, -89.1291) -> (-41.4069, -88.9648)
  line L4132 (-38.5944, -91.6059) -> (-38.7439, -91.8457)
  line L4133 (-39.1361, -92.2504) -> (-39.371, -92.4074)
  line L4134 (-40.7367, -92.6347) -> (-41.0098, -92.5623)
  line L4135 (-40.1737, -92.6612) -> (-40.4561, -92.6679)
  line L4136 (238.499, -90.4718) -> (238.476, -90.6558)
  line L4137 (238.476, -90.6558) -> (238.417, -90.8317)
  line L4138 (238.326, -90.9929) -> (238.205, -91.1333)
  line L4139 (-39.371, -92.4074) -> (-39.6257, -92.5296)
  line L4140 (-36.0238, -90.8735) -> (-35.8793, -90.7573)
  line L4141 (238.205, -91.1333) -> (238.059, -91.2474)
  line L4142 (237.372, -89.5121) -> (237.556, -89.4953)
  line L4143 (236.62, -90.2478) -> (236.676, -90.0711)
  line L4144 (236.866, -91.1052) -> (236.751, -90.9599)
  line L4145 (236.666, -90.795) -> (236.615, -90.6168)
  line L4146 (238.341, -89.9196) -> (238.428, -90.0833)
  line L4147 (97.3362, -89.6177) -> (97.4791, -89.7358)
  line L4148 (237.715, -91.3809) -> (237.53, -91.3951)
  line L4149 (97.5813, -90.9529) -> (97.4601, -91.0932)
  line L4150 (236.766, -89.9086) -> (236.885, -89.7666)
  line L4151 (238.417, -90.8317) -> (238.326, -90.9929)
  line L4152 (96.996, -89.4746) -> (97.1731, -89.5295)
  line L4153 (96.1216, -91.0652) -> (96.0064, -90.9199)
  line L4154 (97.1731, -89.5295) -> (97.3362, -89.6177)
  line L4155 (97.6833, -90.0432) -> (97.7369, -90.2207)
  line L4156 (237.029, -89.6504) -> (237.194, -89.5645)
  line L4157 (97.4791, -89.7358) -> (97.5962, -89.8795)
  line L4158 (236.615, -90.6168) -> (236.6, -90.432)
  line L4159 (236.751, -90.9599) -> (236.666, -90.795)
  line L4160 (237.741, -89.5147) -> (237.918, -89.5695)
  line L4161 (97.6728, -90.7916) -> (97.5813, -90.9529)
  line L4162 (238.481, -90.2608) -> (238.5, -90.4453)
  line L4163 (97.1485, -91.2909) -> (96.9699, -91.3408)
  line L4164 (96.601, -91.3331) -> (96.4246, -91.2758)
  line L4165 (236.6, -90.432) -> (236.62, -90.2478)
  line L4166 (237.346, -91.3731) -> (237.169, -91.3159)
  line L4167 (96.7851, -91.355) -> (96.601, -91.3331)
  line L4168 (238.059, -91.2474) -> (237.893, -91.331)
  line L4169 (237.169, -91.3159) -> (237.007, -91.2254)
  line L4170 (238.428, -90.0833) -> (238.481, -90.2608)
  line L4171 (238.5, -90.4453) -> (238.499, -90.4718)
  line L4172 (238.081, -89.6577) -> (238.224, -89.7759)
  line L4173 (237.53, -91.3951) -> (237.346, -91.3731)
  line L4174 (-35.8793, -90.7573) -> (-35.715, -90.6714)
  line L4175 (-35.715, -90.6714) -> (-35.5371, -90.619)
  line L4176 (237.194, -89.5645) -> (237.372, -89.5121)
  line L4177 (-36.143, -91.0155) -> (-36.0238, -90.8735)
  line L4178 (237.918, -89.5695) -> (238.081, -89.6577)
  line L4179 (97.5962, -89.8795) -> (97.6833, -90.0432)
  line L4180 (238.224, -89.7759) -> (238.341, -89.9196)
  line L4181 (237.893, -91.331) -> (237.715, -91.3809)
  line L4182 (-35.5371, -90.619) -> (-35.3525, -90.6022)
  line L4183 (-35.3525, -90.6022) -> (-35.1681, -90.6216)
  line L4184 (237.007, -91.2254) -> (236.866, -91.1052)
  line L4185 (95.8757, -90.2077) -> (95.9318, -90.031)
  line L4186 (-45.5688, -90.7158) -> (-45.7451, -90.6585)
  line L4187 (96.0211, -89.8685) -> (96.1403, -89.7265)
  line L4188 (96.0064, -90.9199) -> (95.9217, -90.755)
  line L4189 (95.8706, -90.5767) -> (95.8551, -90.392)
  line L4190 (96.8116, -89.4553) -> (96.996, -89.4746)
  line L4191 (-45.0212, -90.6737) -> (-45.1998, -90.7235)
  line L4192 (155.402, -86.8481) -> (155.495, -87.0999)
  line L4193 (-45.7451, -90.6585) -> (-45.9069, -90.568)
  line L4194 (95.8551, -90.392) -> (95.8757, -90.2077)
  line L4195 (155.349, -88.5191) -> (155.207, -88.7468)
  line L4196 (-44.4328, -89.6034) -> (-44.4148, -89.788)
  line L4197 (155.034, -88.9522) -> (154.835, -89.1313)
  line L4198 (154.611, -89.2804) -> (154.369, -89.3966)
  line L4199 (-46.248, -90.1377) -> (-46.2991, -89.9594)
  line L4200 (154.369, -89.3966) -> (154.114, -89.4775)
  line L4201 (153.849, -89.5216) -> (153.58, -89.5279)
  line L4202 (237.556, -89.4953) -> (237.741, -89.5147)
  line L4203 (236.885, -89.7666) -> (237.029, -89.6504)
  line L4204 (97.4601, -91.0932) -> (97.314, -91.2074)
  line L4205 (-45.8849, -88.993) -> (-45.7206, -88.9071)
  line L4206 (154.926, -86.2048) -> (155.115, -86.396)
  line L4207 (155.551, -87.3623) -> (155.57, -87.63)
  line L4208 (-45.1998, -90.7235) -> (-45.3847, -90.7377)
  line L4209 (-45.1737, -88.8574) -> (-44.9966, -88.9122)
  line L4210 (96.4491, -89.5244) -> (96.627, -89.4721)
  line L4211 (155.458, -88.2736) -> (155.349, -88.5191)
  line L4212 (153.58, -89.5279) -> (153.314, -89.4963)
  line L4213 (-44.5735, -89.2622) -> (-44.4864, -89.4259)
  line L4214 (155.531, -88.0153) -> (155.458, -88.2736)
  line L4215 (236.676, -90.0711) -> (236.766, -89.9086)
  line L4216 (97.314, -91.2074) -> (97.1485, -91.2909)
  line L4217 (-46.2991, -89.9594) -> (-46.3147, -89.7747)
  line L4218 (-44.4384, -89.9984) -> (-44.4969, -90.1744)
  line L4219 (-45.9069, -90.568) -> (-46.0481, -90.4479)
  line L4220 (96.2628, -91.1853) -> (96.1216, -91.0652)
  line L4221 (97.7546, -90.4318) -> (97.7314, -90.6157)
  line L4222 (-46.0481, -90.4479) -> (-46.1633, -90.3026)
  line L4223 (-44.4969, -90.1744) -> (-44.5885, -90.3356)
  line L4224 (-44.7096, -90.4759) -> (-44.8557, -90.5901)
  line L4225 (-45.3847, -90.7377) -> (-45.5688, -90.7158)
  line L4226 (-44.4151, -89.8145) -> (-44.4384, -89.9984)
  line L4227 (97.7369, -90.2207) -> (97.755, -90.4052)
  line L4228 (-44.5885, -90.3356) -> (-44.7096, -90.4759)
  line L4229 (153.967, -85.7534) -> (154.229, -85.814)
  line L4230 (95.9217, -90.755) -> (95.8706, -90.5767)
  line L4231 (95.9318, -90.031) -> (96.0211, -89.8685)
  line L4232 (96.2848, -89.6103) -> (96.4491, -89.5244)
  line L4233 (96.627, -89.4721) -> (96.8116, -89.4553)
  line L4234 (-44.8335, -89.0004) -> (-44.6907, -89.1186)
  line L4235 (-44.4864, -89.4259) -> (-44.4328, -89.6034)
  line L4236 (-44.4148, -89.788) -> (-44.4151, -89.8145)
  line L4237 (-44.9966, -88.9122) -> (-44.8335, -89.0004)
  line L4238 (-46.2379, -89.4137) -> (-46.1486, -89.2512)
  line L4239 (-44.6907, -89.1186) -> (-44.5735, -89.2622)
  line L4240 (155.207, -88.7468) -> (155.034, -88.9522)
  line L4241 (155.274, -86.6119) -> (155.402, -86.8481)
  line L4242 (96.1403, -89.7265) -> (96.2848, -89.6103)
  line L4243 (96.9699, -91.3408) -> (96.7851, -91.355)
  line L4244 (-44.8557, -90.5901) -> (-45.0212, -90.6737)
  line L4245 (97.7314, -90.6157) -> (97.6728, -90.7916)
  line L4246 (97.755, -90.4052) -> (97.7546, -90.4318)
  line L4247 (96.4246, -91.2758) -> (96.2628, -91.1853)
  line L4248 (-46.1633, -90.3026) -> (-46.248, -90.1377)
  line L4249 (151.863, -87.0429) -> (151.964, -86.7941)
  line L4250 (155.495, -87.0999) -> (155.551, -87.3623)
  line L4251 (-58.0245, -85.6905) -> (-57.7999, -85.8619)
  line L4252 (-57.6017, -86.0632) -> (-57.4339, -86.2904)
  line L4253 (-57.2019, -86.8041) -> (-57.1425, -87.0803)
  line L4254 (152.099, -86.562) -> (152.265, -86.3513)
  line L4255 (-58.5344, -85.4505) -> (-58.271, -85.5524)
  line L4256 (155.566, -87.7493) -> (155.531, -88.0153)
  line L4257 (151.771, -87.5703) -> (151.798, -87.3033)
  line L4258 (152.265, -86.3513) -> (152.459, -86.166)
  line L4259 (-57.1425, -87.0803) -> (-57.1225, -87.3621)
  line L4260 (152.915, -85.8863) -> (153.169, -85.7973)
  line L4261 (152.369, -89.015) -> (152.187, -88.818)
  line L4262 (154.479, -85.9108) -> (154.713, -86.042)
  line L4263 (151.798, -87.3033) -> (151.863, -87.0429)
  line L4264 (153.314, -89.4963) -> (153.055, -89.4276)
  line L4265 (-57.1265, -87.4877) -> (-57.1641, -87.7677)
  line L4266 (154.229, -85.814) -> (154.479, -85.9108)
  line L4267 (-57.1225, -87.3621) -> (-57.1265, -87.4877)
  line L4268 (-60.844, -88.3802) -> (-60.9703, -88.1275)
  line L4269 (-45.7206, -88.9071) -> (-45.5428, -88.8548)
  line L4270 (155.115, -86.396) -> (155.274, -86.6119)
  line L4271 (151.781, -87.8385) -> (151.771, -87.5703)
  line L4272 (-57.6863, -88.7539) -> (-57.8967, -88.9424)
  line L4273 (-60.9703, -88.1275) -> (-61.0597, -87.8595)
  line L4274 (-45.5428, -88.8548) -> (-45.3581, -88.838)
  line L4275 (-46.3147, -89.7747) -> (-46.294, -89.5904)
  line L4276 (-46.1486, -89.2512) -> (-46.0294, -89.1092)
  line L4277 (-46.0294, -89.1092) -> (-45.8849, -88.993)
  line L4278 (152.459, -86.166) -> (152.677, -86.01)
  line L4279 (151.915, -88.3571) -> (151.83, -88.1025)
  line L4280 (-57.355, -88.298) -> (-57.5045, -88.5377)
  line L4281 (-59.4973, -89.3267) -> (-59.7704, -89.2543)
  line L4282 (-61.0597, -87.8595) -> (-61.1104, -87.5816)
  line L4283 (-61.1104, -87.5816) -> (-61.1215, -87.2993)
  line L4284 (152.807, -89.3229) -> (152.577, -89.1845)
  line L4285 (153.432, -85.745) -> (153.7, -85.7302)
  line L4286 (154.114, -89.4775) -> (153.849, -89.5216)
  line L4287 (-58.8097, -85.3867) -> (-58.5344, -85.4505)
  line L4288 (152.677, -86.01) -> (152.915, -85.8863)
  line L4289 (-46.294, -89.5904) -> (-46.2379, -89.4137)
  line L4290 (-57.7999, -85.8619) -> (-57.6017, -86.0632)
  line L4291 (-57.4339, -86.2904) -> (-57.2997, -86.5391)
  line L4292 (-57.2997, -86.5391) -> (-57.2019, -86.8041)
  line L4293 (153.169, -85.7973) -> (153.432, -85.745)
  line L4294 (153.7, -85.7302) -> (153.967, -85.7534)
  line L4295 (154.713, -86.042) -> (154.926, -86.2048)
  line L4296 (153.055, -89.4276) -> (152.807, -89.3229)
  line L4297 (152.187, -88.818) -> (152.035, -88.5972)
  line L4298 (-59.7704, -89.2543) -> (-60.0305, -89.1441)
  line L4299 (-57.2408, -88.0396) -> (-57.355, -88.298)
  line L4300 (-61.1215, -87.2993) -> (-61.0927, -87.0182)
  line L4301 (-57.5045, -88.5377) -> (-57.6863, -88.7539)
  line L4302 (152.577, -89.1845) -> (152.369, -89.015)
  line L4303 (-61.0927, -87.0182) -> (-61.0246, -86.7441)
  line L4304 (-60.9186, -86.4822) -> (-60.7767, -86.2379)
  line L4305 (155.57, -87.63) -> (155.566, -87.7493)
  line L4306 (-60.6834, -88.6126) -> (-60.844, -88.3802)
  line L4307 (151.83, -88.1025) -> (151.781, -87.8385)
  line L4308 (151.964, -86.7941) -> (152.099, -86.562)
  line L4309 (-58.271, -85.5524) -> (-58.0245, -85.6905)
  line L4310 (-45.3581, -88.838) -> (-45.1737, -88.8574)
  line L4311 (152.035, -88.5972) -> (151.915, -88.3571)
  line L4312 (154.835, -89.1313) -> (154.611, -89.2804)
  line L4313 (179.985, -89.0689) -> (179.755, -88.9305)
  line L4314 (-59.6503, -85.433) -> (-59.3732, -85.3779)
  line L4315 (-60.3974, -85.8211) -> (-60.1675, -85.6568)
  line L4316 (179.755, -88.9305) -> (179.547, -88.761)
  line L4317 (182.748, -87.376) -> (182.744, -87.4953)
  line L4318 (180.233, -89.1736) -> (179.985, -89.0689)
  line L4319 (180.492, -89.2423) -> (180.233, -89.1736)
  line L4320 (181.145, -85.4994) -> (181.407, -85.56)
  line L4321 (-58.6556, -89.3068) -> (-58.9343, -89.3532)
  line L4322 (179.547, -88.761) -> (179.365, -88.564)
  line L4323 (180.758, -89.2739) -> (180.492, -89.2423)
  line L4324 (-57.1641, -87.7677) -> (-57.2408, -88.0396)
  line L4325 (-59.0911, -85.3623) -> (-58.8097, -85.3867)
  line L4326 (179.855, -85.756) -> (180.093, -85.6323)
  line L4327 (181.027, -89.2676) -> (180.758, -89.2739)
  line L4328 (179.365, -88.564) -> (179.213, -88.3432)
  line L4329 (179.093, -88.1031) -> (179.008, -87.8485)
  line L4330 (180.878, -85.4762) -> (181.145, -85.4994)
  line L4331 (179.443, -86.0973) -> (179.637, -85.912)
  line L4332 (-53.3434, -88.7918) -> (-53.4646, -88.9322)
  line L4333 (178.959, -87.5845) -> (178.949, -87.3163)
  line L4334 (180.61, -85.491) -> (180.878, -85.4762)
  line L4335 (179.041, -86.7889) -> (179.142, -86.5401)
  line L4336 (-59.3732, -85.3779) -> (-59.0911, -85.3623)
  line L4337 (181.407, -85.56) -> (181.657, -85.6568)
  line L4338 (-60.0305, -89.1441) -> (-60.2725, -88.9984)
  line L4339 (179.008, -87.8485) -> (178.959, -87.5845)
  line L4340 (179.142, -86.5401) -> (179.277, -86.308)
  line L4341 (-60.7767, -86.2379) -> (-60.6018, -86.0161)
  line L4342 (182.104, -85.9508) -> (182.293, -86.142)
  line L4343 (182.729, -87.1083) -> (182.748, -87.376)
  line L4344 (-60.1675, -85.6568) -> (-59.9168, -85.5266)